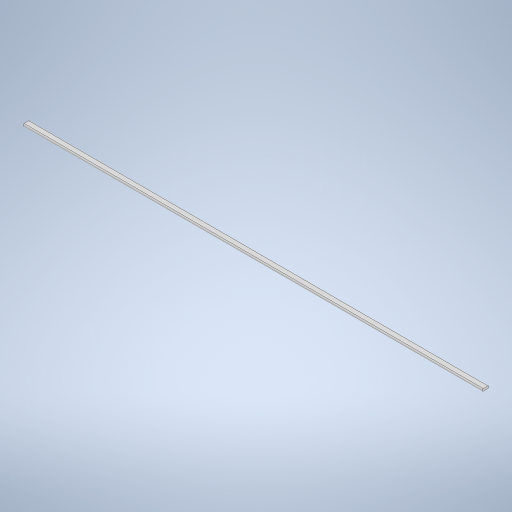
# Autodesk Inventor part: Hot Pipe
Saved by Autodesk Inventor 2024 (Build 280153000, 153)
## iProperties
Created: 2023-06-24
Part Number: Hot Pipe
Material: 常规
Document SubType Name: Sheet Metal
Designer: lunima
Density: 1 g/cm^3
Sheet Metal Rule: 默认_mm
Appearance: 默认
Author: lunima
Autodesk Inventor part; units mm, degrees
ref_plane "YZ Plane" through (0, 0, 0) normal (1, 0, 0) x (0, 1, 0)
ref_plane "XZ Plane" through (0, 0, 0) normal (0, 1, 0) x (-1, 0, 0)
ref_plane "XY Plane" through (0, 0, 0) normal (0, 0, 1) x (1, 0, 0)
sketch "草图1" plane through (0, 0, 0) normal (1, 0, 0) x (0, 1, 0)
  line L0 (0, 0) -> (0, -3) construction
  line L1 (-0.75, 0) -> (-0.75, -3)
  line L2 (0.75, -3) -> (0.75, 0)
  arc A0 (0.75, 0) -> (-0.75, 0) centre (0, 0) ccw
  arc A1 (-0.75, -3) -> (0.75, -3) centre (0, -3) ccw
  point P0 (0, -1.5)
  dimension "d0" = 3
  dimension "d1" = 1.5
  constraints: 8 end point, 4 point on circle, 4 tangent, 2 centre point, 1 midpoint, 1 parallel, 1 vertical
  measures "d0" distance of L0.start L0.end
  measures "d1" diameter of A1
sketch "草图2" plane through (0, 0, 0) normal (1, 0, 0) x (0, 1, 0)
  point P0 (0, 0)
extrude "拉伸1" add sketch "草图1" along normal blind 300
equation "\"折弯半径\" = 厚度"
equation "\"折弯释压宽度\" = 厚度"
equation "\"折弯释压深度\" = 0.5 * 厚度"
equation "\"拐角释压尺寸\" = 4 * 厚度"
equation "\"最小余量\" = 2 * 厚度"
equation "\"过渡半径\" = 折弯半径"
equation "\"Jacobi半径尺寸\" = 折弯半径"
equation "\"间隙大小\" = 厚度"
equation "\"厚度\" = 0.5"
